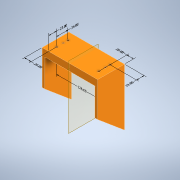
# Autodesk Inventor part: bracketForGarageLowerHalf
Saved by Autodesk Inventor 2022.2 (Build 262287000, 287)
## iProperties
Created: 2021-10-20
Part Number: bracketForGarageLowerHalf
Material: PC/ABS Plastic
Document SubType Name: Modeling
Designer: robst
Density: 0.357273 g/cm^3
Appearance: Orange
Author: robst
Autodesk Inventor part; units mm, degrees
note: some values were not read from the file. Chosen so that the rebuilt part matches the saved one: direction of "HoleForLeftSideOf2x4"; direction of "HolesForRightSideOf2x4".
ref_plane "XZ Plane" through (0, 0, 0) normal (0, 1, 0) x (-1, 0, 0)
ref_plane "XY Plane" through (0, 0, 0) normal (0, 0, 1) x (1, 0, 0)
sketch "Sketch8" plane through (0, 0, 0) normal (0, 1, 0) x (-1, 0, 0)
  line L0 (83, 40) -> (-83, 40)
  line L1 (-83, 40) -> (-83, -40)
  line L2 (-83, -40) -> (83, -40)
  line L3 (83, -40) -> (83, 40)
  line L4 (83, 40) -> (-83, -40) construction
  line L5 (-83, 40) -> (83, -40) construction
  point P0 (0, 0)
  dimension "d28" = 80
  dimension "d29" = 166
  constraints: 12 end point, 2 midpoint, 2 parallel, 1 horizontal, 1 perpendicular
  measures "d28" distance of L2.end L0.start
  measures "d29" distance between parallel lines of L1 L3
extrude "Extrusion8" add sketch "Sketch8" against normal blind 8
sketch "Sketch9" plane through (0, -8, 0) normal (0, -1, 0) x (1, 0, 0)
  line L0 (83, 40) -> (-83, 40) projected
  line L1 (-83, -40) -> (83, -40) projected
  line L2 (-83, 40) -> (-75, 40)
  line L3 (-75, 40) -> (-75, -40)
  line L4 (-75, -40) -> (-83, -40)
  line L5 (-83, -40) -> (-83, 40)
  line L6 (83, -40) -> (83, 40) projected
  line L7 (83, -40) -> (75, -40)
  line L8 (75, -40) -> (75, 40)
  line L9 (75, 40) -> (83, 40)
  line L10 (83, 40) -> (83, -40)
  point P0 (0, 0)
  point P1 (75, 40)
  point P2 (75, -40)
  dimension "d32" = 8
  dimension "d33" = 8
  constraints: 16 end point, 4 parallel, 2 horizontal, 2 perpendicular, 2 point on line
  measures "d32" distance between parallel lines of L3 L5
  measures "d33" distance between parallel lines of L6 L8
extrude "armsForCameraCase" add sketch "Sketch9" along normal blind 150 contours L6 L1 L8 L0 | L3 L1 L5 L0
sketch "Sketch10" plane through (-75, -8, 40) normal (1, 0, 0) x (0, 0, -1)
  line L0 (0, 0) -> (80, 0) projected
  line L1 (80, 0) -> (80, -150) projected
  line L2 (80, -150) -> (0, -150) projected
  line L3 (0, 0) -> (0, -150) projected
  line L4 (0, 0) -> (80, -67.128)
  line L5 (80, -67.128) -> (80, 0)
  line L6 (80, 0) -> (0, 0)
  point P0 (40, 8)
  point P1 (40, -33.564)
  dimension "d48" = 40
  constraints: 6 end point, 2 collinear, 1 midpoint, 1 point on line
  measures "d48" angle of L4 L0
extrude "Extrusion10" add sketch "Sketch10" along normal up to surface (150 mm away) contours L0 L1 L4
sketch "Sketch11" plane through (0, 0, 0) normal (0, 1, 0) x (1, 0, 0)
  line L0 (83, 40) -> (-83, 40) projected
  line L1 (-83, -40) -> (83, -40) projected
  line L2 (-83, 40) -> (-83, -40) projected
  line L3 (83, -40) -> (83, 40) projected
  line L4 (-31.038, -40) -> (-9.602, 40)
  line L5 (-9.602, 40) -> (-17.8842, 40)
  line L6 (-75, 40) -> (75, 40) projected
  line L7 (-17.8842, 40) -> (-39.3202, -40)
  line L8 (-39.3202, -40) -> (-31.038, -40)
  line L9 (-31.038, -40) -> (-31.038, 40) construction
  line L10 (0, -40) -> (0, 40) construction
  line L11 (9.602, -40) -> (31.038, 40)
  line L12 (31.038, 40) -> (39.3202, 40)
  line L13 (39.3202, 40) -> (17.8842, -40)
  line L14 (17.8842, -40) -> (9.602, -40)
  point P0 (0, 0)
  point P1 (0, -40)
  point P2 (0, -40)
  point P3 (-20.32, 0)
  point P4 (0, 0)
  point P5 (20.32, 0)
  point P6 (39.3202, 40)
  point P7 (31.038, 40)
  point P8 (-17.8842, 40)
  dimension "d39" = -15
  dimension "d40" = 8
  dimension "d42" = 8
  dimension "d44" = 20.32
  dimension "d45" = 20.32
  constraints: 20 end point, 5 point on line, 4 midpoint, 3 parallel, 2 horizontal, 1 perpendicular, 8 other
  measures "d39" angle of L4 L9
  measures "d40" distance between parallel lines of L7 L4
  measures "d42" distance between parallel lines of L13 L11
  measures "d44" distance of point (-20.32, 0) point (0, 0)
  measures "d45" distance of point (20.32, 0) point (0, 0)
extrude "Extrusion11" add sketch "Sketch11" along normal blind 104.1375 contours L13 L1 L11 L0 | L4 L1 L7 L0
sketch "Sketch12" plane through (0, 0, 0) normal (0, 1, 0) x (1, 0, 0)
  line L0 (31.038, 40) -> (-9.602, 40) projected
  line L1 (31.038, 40) -> (9.602, -40) projected
  line L2 (-31.038, -40) -> (9.602, -40) projected
  line L3 (-31.038, -40) -> (-9.602, 40) projected
  line L4 (-9.602, 40) -> (31.038, 40)
  line L5 (31.038, 40) -> (9.602, -40)
  line L6 (9.602, -40) -> (-31.038, -40)
  line L7 (-9.602, 40) -> (-31.038, -40) projected
  line L8 (-31.038, -40) -> (-9.602, 40)
  point P0 (0, 0)
  constraints: 8 end point, 3 equal length
extrude "Extrusion12" add sketch "Sketch12" along normal blind 20
sketch "Sketch13" plane through (-83, 0, -40) normal (-1, 0, 0) x (0, 0, 1)
  line L0 (0, -75.128) -> (80, -8) projected
  line L1 (80, 0) -> (80, -158) projected
  line L2 (80, -158) -> (0, -158) projected
  line L3 (0, 0) -> (0, -158) projected
  line L4 (80, -158) -> (0, -158) construction
  line L5 (40, -158) -> (40, -41.564) construction
  line L6 (80, -8) -> (0, -75.128) construction
  line L7 (0, -205.6687) -> (80, -138.5407) construction
  line L8 (80, -8) -> (80, -158) construction
  point P0 (40, 0)
  point P1 (40, -172.1047)
  point P2 (20, -188.8867)
  point P3 (60, -155.3227)
  dimension "centerForTwoHoles" = 26.1081
  dimension "d51" = 100
  dimension "diagonalLine" = 104.4326
  dimension "d62" = 26.1081
  dimension "d63" = 26.1081
  constraints: 4 end point, 4 point on line, 3 midpoint, 1 parallel
  measures "d51" distance between parallel lines of L7 L0
  measures "diagonalLine" distance of L7.start L7.end
  measures "d62" distance of point (20, -188.887) L7.start
  measures "d63" distance of point (60, -155.323) L7.end
hole "HolesForAttchingToLowerCase" at (-83, -172.1047, 0) at (-83, -188.8867, -20) at (-83, -155.3227, 20) direction (1, 0, 0) diameter 6.7564 end through all clearance for "Hex Machine Screw" size "1/4" standard "Ansi Unified Screw Threads"
sketch "Sketch14" plane through (-83, 0, -40) normal (-1, 0, 0) x (0, 0, 1)
  line L0 (80, 0) -> (80, -158) projected
  line L1 (80, -158) -> (0, -158) projected
  line L2 (0, 0) -> (0, -158) projected
  line L3 (0, -75.128) -> (80, -8) projected
  line L4 (0, -75.128) -> (0, -158) projected
  line L5 (0, -158) -> (80, -90.872)
  line L6 (0, -158) -> (80, -158) projected
  line L7 (0, -158) -> (80, -158)
  line L8 (80, -158) -> (80, -90.872)
  point P0 (40, 0)
  constraints: 6 end point, 2 collinear, 1 parallel, 1 point on line
extrude "Extrusion13" cut sketch "Sketch14" against normal through all contours L0 L1 L5
sketch "Sketch15" plane through (-39.3202, 0, 40) normal (-0.9659258, 0, -0.258819) x (-0.258819, 0, 0.9659258)
  line L0 (-82.8221, 104.1375) -> (0, 104.1375) projected
  line L1 (0, 0) -> (0, 104.1375) projected
  line L2 (-82.8221, 0) -> (-82.8221, 104.1375) projected
  line L3 (-2.1436, 20) -> (-84.9657, 20) projected
  line L4 (-82.8221, 40) -> (0, 40) construction
  line L5 (-57.8221, 40) -> (-57.8221, 104.1375) construction
  point P0 (-48.8138, 0)
  point P1 (-82.8221, 52.0688)
  point P2 (-37.8221, 40)
  point P3 (-17.8221, 40)
  point P4 (-57.8221, 60)
  point P5 (-37.8221, 60)
  point P6 (-17.8221, 60)
  point P7 (-57.8221, 80)
  point P8 (-37.8221, 80)
  point P9 (-17.8221, 80)
  dimension "d64" = 25
  dimension "d74" = 20
  dimension "d77" = 20
  dimension "d90" = 20
  constraints: 4 end point, 4 point on line, 2 perpendicular, 1 coincident, 1 horizontal, 1 midpoint, 1 vertical, 8 other
  measures "d64" distance from line of point (-82.822, 52.069) L5
  measures "d74" distance of point (-57.822, 40) point (-37.822, 40)
  measures "d77" distance of point (-57.822, 40) point (-57.822, 60)
  measures "d90" distance between parallel lines of L4 L3
hole "HoleForLeftSideOf2x4" at (-24.3547, 40, -15.8519) at (-29.5311, 40, 3.4667) at (-34.7075, 40, 22.7852) at (-29.5311, 60, 3.4667) at (-24.3547, 60, -15.8519) at (-34.7075, 60, 22.7852) at (-34.7075, 80, 22.7852) at (-29.5311, 80, 3.4667) at (-24.3547, 80, -15.8519) direction (0.9659258, 0, 0.258819) diameter 4.496 depth 8 countersink diameter 8.433 countersink angle 82 clearance for "Flat Head Machine Screw (82)" size "#8" standard "Ansi Unified Screw Threads"
sketch "Sketch16" plane through (39.3202, 0, -40) normal (0.9659258, 0, 0.258819) x (0.258819, 0, -0.9659258)
  line L0 (-82.8221, 104.1375) -> (0, 104.1375) projected
  line L1 (0, 0) -> (0, 104.1375) projected
  line L2 (-82.8221, 0) -> (-82.8221, 104.1375) projected
  line L3 (-82.8221, 0) -> (-65.9689, 0) projected
  line L4 (-2.1436, 20) -> (-84.9657, 20) projected
  line L5 (-82.8221, 40) -> (0, 40) construction
  line L6 (-67.8221, 40) -> (-67.8221, 104.1375) construction
  point P0 (-48.8138, 0)
  point P1 (-47.8221, 40)
  point P2 (-27.8221, 40)
  point P3 (-67.8221, 60)
  point P4 (-47.8221, 60)
  point P5 (-27.8221, 60)
  point P6 (-67.8221, 80)
  point P7 (-47.8221, 80)
  point P8 (-27.8221, 80)
  dimension "d80" = 20
  dimension "d81" = 15
  dimension "d84" = 20
  dimension "d87" = 20
  constraints: 4 end point, 4 point on line, 2 perpendicular, 1 coincident, 1 horizontal, 1 vertical, 8 other
  measures "d80" distance between parallel lines of L5 L4
  measures "d81" distance between parallel lines of L6 L2
  measures "d84" distance of point (-67.822, 40) point (-47.822, 40)
  measures "d87" distance of point (-67.822, 40) point (-67.822, 60)
hole "HolesForRightSideOf2x4" at (26.9429, 40, 6.1926) at (32.1193, 40, -13.1259) at (21.7665, 60, 25.5111) at (26.9429, 60, 6.1926) at (32.1193, 60, -13.1259) at (21.7665, 80, 25.5111) at (26.9429, 80, 6.1926) at (32.1193, 80, -13.1259) at (21.7665, 40, 25.5111) direction (-0.9659258, 0, -0.258819) diameter 4.496 depth 8 countersink diameter 8.433 countersink angle 82 clearance for "Flat Head Machine Screw (82)" size "#8" standard "Ansi Unified Screw Threads"
sketch "Sketch17" plane through (0, 20, 0) normal (0, 1, 0) x (1, 0, 0)
  line L0 (31.038, 40) -> (9.602, -40) projected
  line L1 (-31.038, -40) -> (9.602, -40) projected
  line L2 (-31.038, -40) -> (-9.602, 40) projected
  line L3 (31.038, 40) -> (-9.602, 40) projected
  line L4 (20.6122, 32) -> (3.4634, -32)
  line L5 (3.4634, -32) -> (-20.6122, -32)
  line L6 (-20.6122, -32) -> (-3.4634, 32)
  line L7 (-3.4634, 32) -> (20.6122, 32)
  point P0 (0, 0)
  point P1 (10.718, 40)
  point P2 (-8.5744, -32)
  dimension "d98" = 8
  dimension "d99" = 8
  dimension "d101" = 8
  dimension "d102" = 8
  constraints: 8 end point, 4 parallel, 2 midpoint, 1 horizontal
  measures "d98" distance between parallel lines of L4 L0
  measures "d99" distance between parallel lines of L6 L2
  measures "d101" distance from line of point (10.718, 40) L7
  measures "d102" distance from line of point (-8.574, -32) L1
extrude "Extrusion14" cut sketch "Sketch17" against normal through all contours L4 L5 L6 L7
sketch "Sketch18" plane through (0, 0, 0) normal (0, 1, 0) x (1, 0, 0)
  line L0 (17.8842, -40) -> (83, -40) projected
  line L1 (17.8842, -40) -> (39.3202, 40) projected
  line L2 (83, 40) -> (39.3202, 40) projected
  line L3 (83, -40) -> (83, 40) projected
  line L4 (67, -32) -> (67, 32)
  line L5 (67, 32) -> (45.4588, 32)
  line L6 (45.4588, 32) -> (28.31, -32)
  line L7 (28.31, -32) -> (67, -32)
  line L8 (39.3202, 40) -> (17.8842, -40) projected
  line L9 (17.8842, -40) -> (83, -40) projected
  line L10 (83, -40) -> (83, 40) projected
  line L11 (83, 40) -> (39.3202, 40) projected
  point P0 (0, 0)
  dimension "d105" = 8
  dimension "d107" = 8
  dimension "d108" = 16
  dimension "d109" = 8
  constraints: 8 end point, 4 parallel, 1 perpendicular
  measures "d105" distance between parallel lines of L7 L0
  measures "d107" distance between parallel lines of L1 L6
  measures "d108" distance between parallel lines of L3 L4
  measures "d109" distance between parallel lines of L5 L2
extrude "Extrusion15" cut sketch "Sketch18" against normal through all contours L7 L6 L5 L4
sketch "Sketch19" plane through (0, 0, 0) normal (0, 1, 0) x (1, 0, 0)
  line L0 (-17.8842, 40) -> (-39.3202, -40) projected
  line L1 (-83, -40) -> (-39.3202, -40) projected
  line L2 (-83, 40) -> (-83, -40) projected
  line L3 (-17.8842, 40) -> (-83, 40) projected
  line L4 (-28.31, 32) -> (-45.4588, -32)
  line L5 (-45.4588, -32) -> (-67, -32)
  line L6 (-67, -32) -> (-67, 32)
  line L7 (-67, 32) -> (-28.31, 32)
  point P0 (0, 0)
  point P1 (-61.1601, -40)
  dimension "d112" = 8
  dimension "d113" = 16
  dimension "d114" = 8
  dimension "d115" = 8
  constraints: 8 end point, 4 parallel, 1 horizontal, 1 midpoint
  measures "d112" distance between parallel lines of L0 L4
  measures "d113" distance between parallel lines of L6 L2
  measures "d114" distance from line of point (-61.16, -40) L5
  measures "d115" distance between parallel lines of L3 L7
extrude "Extrusion16" cut sketch "Sketch19" against normal through all contours L4 L5 L6 L7
sketch "Sketch27" plane through (-75, -8, 40) normal (0, 0, 1) x (1, 0, 0)
  line L0 (92.8842, 8) -> (158, 8) projected
  line L1 (92.8842, 8) -> (92.8842, 112.1375) projected
  line L2 (158, 8) -> (158, -82.872) projected
  line L3 (92.8842, 38) -> (158, 8)
  line L4 (158, 8) -> (92.8842, 8)
  line L5 (92.8842, 8) -> (92.8842, 38)
  point P0 (75, 8)
  dimension "d152" = 30
  constraints: 6 end point, 2 collinear, 1 point on line
  measures "d152" distance of L0.start L3.start
sketch "Sketch28" plane through (67, 0, 32) normal (0, 0, -1) x (-1, 0, 0)
  line L0 (-16, 0) -> (47.9394, 0)
  line L1 (49.1158, 0) -> (49.1158, 104.1375) projected
  line L2 (47.9394, 0) -> (47.9394, 30)
  line L3 (47.9394, 30) -> (-16, 0)
  point P0 (67, 0)
  dimension "d153" = 30
  constraints: 6 end point, 1 parallel, 1 perpendicular
  measures "d153" distance of L0.end L2.end
loft "Loft5" add profiles "Sketch27", "Sketch28"
sketch "Sketch29" plane through (75, -75.128, -40) normal (0, 0, -1) x (-1, 0, 0)
  line L0 (-8, 75.128) -> (35.6798, 75.128) projected
  line L1 (35.6798, 75.128) -> (35.6798, 179.2655) projected
  line L2 (-8, 75.128) -> (-8, -15.7441) projected
  line L3 (-8, 75.128) -> (35.6798, 75.128)
  line L4 (35.6798, 75.128) -> (35.6798, 105.128)
  line L5 (35.6798, 105.128) -> (-8, 75.128)
  point P0 (75, 75.128)
  dimension "d158" = 30
  constraints: 6 end point, 1 collinear, 1 point on line
  measures "d158" distance of L4.end L0.end
sketch "Sketch30" plane through (45.4588, 0, -32) normal (0, 0, 1) x (1, 0, 0)
  line L0 (-6.1386, 0) -> (-6.1386, 104.1375) projected
  line L1 (37.5412, 0) -> (-6.1386, 0) projected
  line L2 (-6.1386, 0) -> (-6.1386, 104.1375) projected
  line L3 (-6.1386, 0) -> (37.5412, 0)
  line L4 (37.5412, 0) -> (-6.1386, 30)
  line L5 (-6.1386, 30) -> (-6.1386, 0)
  point P0 (-45.4588, 0)
  dimension "d159" = 30
  constraints: 6 end point, 1 collinear, 1 perpendicular, 1 point on line
  measures "d159" distance of L4.end L0.start
loft "Loft6" add profiles "Sketch29", "Sketch30"
sketch "Sketch31" plane through (-75, -8, 40) normal (0, 0, 1) x (1, 0, 0)
  line L0 (-8, 8) -> (35.6798, 8) projected
  line L1 (35.6798, 8) -> (35.6798, 112.1375) projected
  line L2 (57.1158, 8) -> (-8, 8) projected
  line L3 (-8, 8) -> (35.6798, 8)
  line L4 (35.6798, 8) -> (35.6798, 47)
  line L5 (35.6798, 47) -> (-8, 8)
  point P0 (75, 8)
  dimension "d164" = 39
  constraints: 6 end point, 1 horizontal, 1 point on line
  measures "d164" distance of L4.end L0.end
sketch "Sketch32" plane through (-45.4588, 0, 32) normal (0, 0, -1) x (-1, 0, 0)
  line L0 (37.5412, 0) -> (-6.1386, 0) projected
  line L1 (37.5412, 0) -> (-8.7458, 0)
  line L2 (-8.7458, 0) -> (-8.7458, 30)
  line L3 (-8.7458, 30) -> (37.5412, 0)
  point P0 (-45.4588, 0)
  dimension "d165" = 30
  constraints: 6 end point, 1 horizontal, 1 perpendicular
  measures "d165" distance of L1.end L2.end
loft "Loft7" add profiles "Sketch31", "Sketch32"
sketch "Sketch33" plane through (75, -75.128, -40) normal (0, 0, -1) x (-1, 0, 0)
  line L0 (92.8842, 75.128) -> (158, 75.128) projected
  line L1 (92.8842, 75.128) -> (92.8842, 179.2655) projected
  line L2 (112.1766, 75.128) -> (92.8842, 75.128) projected
  line L3 (92.8842, 75.128) -> (158, 75.128)
  line L4 (158, 75.128) -> (92.8842, 105.128)
  line L5 (92.8842, 105.128) -> (92.8842, 75.128)
  point P0 (75, 75.128)
  dimension "d171" = 30
  constraints: 6 end point, 2 collinear, 1 point on line
  measures "d171" distance of L4.end L0.start
sketch "Sketch34" plane through (-67, 0, -32) normal (0, 0, 1) x (1, 0, 0)
  line L0 (49.1158, 0) -> (-16, 0) projected
  line L1 (49.1158, 0) -> (49.1158, 104.1375) projected
  line L2 (-16, 0) -> (50.0262, 0)
  line L3 (29.8234, 0) -> (49.1158, 0) projected
  line L4 (50.0262, 0) -> (50.0262, 30)
  line L5 (50.0262, 30) -> (-16, 0)
  point P0 (67, 0)
  dimension "d170" = 30
  constraints: 6 end point, 1 point on line, 1 vertical
  measures "d170" distance of L2.end L4.end
loft "Loft8" add profiles "Sketch33", "Sketch34"
split "Split3" plane through (0, 0, 0) removes the side toward (0, 1, 0)
sketch "Sketch37" plane through (0, 0, 0) normal (0, 1, 0) x (1, 0, 0)
  line L0 (-83, 40) -> (83, 40) projected
  line L1 (83, -40) -> (83, 40) projected
  line L2 (83, -40) -> (-83, -40) projected
  line L3 (-83, 40) -> (-83, -40) projected
  line L4 (-82, -40) -> (82, -40)
  line L5 (82, -40) -> (82, 40)
  line L6 (82, 40) -> (-82, 40)
  line L7 (-82, 40) -> (-82, -40)
  line L8 (-82, -40) -> (82, 40) construction
  line L9 (82, -40) -> (-82, 40) construction
  point P0 (0, 0)
  constraints: 12 end point, 2 midpoint, 2 parallel, 1 perpendicular
extrude "ExtrusionForMatingUpperHalf" add sketch "Sketch37" along normal blind 12.5
sketch "Sketch38" plane through (0, 0, 0) normal (0, -1, 0) x (1, 0, 0)
  point P0 (-63, -17)
  point P1 (63, -17)
  point P2 (63, 17)
  point P3 (-63, 17)
hole "HoleForNumber10Screws" at (-63, 0, -17) at (63, 0, -17) at (63, 0, 17) at (-63, 0, 17) direction (0, 1, 0) diameter 5.1054 end through all
sketch "SketchForHeatSetInserts" plane through (0, 12.5, 0) normal (0, 1, 0) x (1, 0, 0)
  circle A0 centre (-63, 17) radius 2.5527 construction
  circle A1 centre (63, -17) radius 2.5527 construction
  line L0 (-63, 17) -> (63, 17) construction
  line L1 (63, 17) -> (63, -17) construction
  line L2 (63, -17) -> (-63, -17) construction
  line L3 (-63, -17) -> (-63, 17) construction
  circle A2 centre (63, 17) radius 2.5527 projected
  point P0 (0, 0)
  constraints: 8 end point, 4 coincident, 2 parallel, 1 horizontal, 1 perpendicular
hole "HoleForInserts" at (-63, 12.5, -17) at (63, 12.5, -17) at (63, 12.5, 17) at (-63, 12.5, 17) direction (0, -1, 0) diameter 6.32 depth 9.525 counterbore diameter 6.5278 counterbore depth 7.41
sketch "Sketch42" plane through (-75, -8, 40) normal (0, -0.7660444, 0.6427876) x (1, 0, 0)
  line L0 (-8, 13.1771) -> (158, 13.1771) projected
  line L1 (0, -104.4326) -> (150, -104.4326) projected
  ellipse E0 centre (138, -12.4767) end of major axis (140.5527, -12.4767) minor radius 1.9555 projected
  ellipse E1 centre (138, -38.5222) end of major axis (140.5527, -38.5222) minor radius 1.9555 projected
  ellipse E2 centre (12, -12.4767) end of major axis (14.5527, -12.4767) minor radius 1.9555 projected
  ellipse E3 centre (12, -38.5222) end of major axis (14.5527, -38.5222) minor radius 1.9555 projected
  line L2 (138, 13.1771) -> (138, -104.4326) construction
  line L3 (12, 13.1771) -> (12, -104.4326) construction
  point P0 (75, -25.4995)
  point P1 (138, -20.0649)
  point P2 (12, -20.0649)
  dimension "d210" = 33.242
  dimension "d211" = 33.242
  constraints: 6 point on line, 4 end point, 2 perpendicular
  measures "d210" distance from line of L0 point (12, -20.065)
  measures "d211" distance from line of point (138, -20.065) L0
hole "Hole8" at (63, -20.8974, 24.6294) at (-63, -20.8974, 24.6294) direction (0, 0.7660444, -0.6427876) diameter 5.1054 depth 50 clearance for "Hex Machine Screw" size "#10" standard "Ansi Unified Screw Threads"
equation "\"d28\" = widthOfBracket"
equation "\"d30\" = wallThickness"
equation "\"d32\" = wallThickness"
equation "\"d33\" = wallThickness"
equation "\"d48\" = elevation"
equation "\"d39\" = azimuth"
equation "\"d40\" = wallThickness"
equation "\"d42\" = wallThickness"
equation "\"d44\" = 0.5 * twoByFourWidth"
equation "\"d45\" = 0.5 * twoByFourWidth"
equation "\"d46\" = twoByFourDepth + baseBelowTwoByFour"
equation "\"d49\" = baseBelowTwoByFour"
equation "\"centerForTwoHoles\" = 0.25 * diagonalLine"
equation "\"d62\" = centerForTwoHoles"
equation "\"d63\" = centerForTwoHoles"
equation "\"d98\" = wallThickness"
equation "\"d99\" = wallThickness"
equation "\"d101\" = wallThickness"
equation "\"d102\" = wallThickness"
equation "\"d105\" = wallThickness"
equation "\"d107\" = wallThickness"
equation "\"d108\" = 2 * wallThickness"
equation "\"d109\" = wallThickness"
equation "\"d112\" = wallThickness"
equation "\"d113\" = 2 * wallThickness"
equation "\"d114\" = wallThickness"
equation "\"d115\" = wallThickness"
equation "\"d185\" = depthOfExtrusionForMatingUpperHalf"
equation "\"wallThickness\" = 8"
equation "\"widthOfBracket\" = 80"
equation "\"twoByFourWidth\" = 40.64"
equation "\"twoByFourDepth\" = 84.1375"
equation "\"azimuth\" = -15deg"
equation "\"elevation\" = 40deg"
equation "\"baseBelowTwoByFour\" = 20"
equation "\"depthOfExtrusionForMatingUpperHalf\" = 12.5"
equation "\"topWallThickness\" = 12.7"
body "Solid2"
